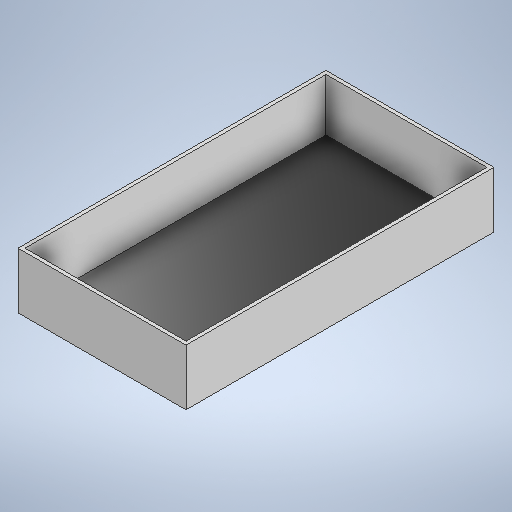
# Autodesk Inventor part: Blackout Box
Saved by Autodesk Inventor 2025 (Build 290162000, 162)
## iProperties
Created: 2024-06-19
Part Number: Blackout Box
Material: Generic
Document SubType Name: Modeling
Designer: User
Density: 1 g/cm^3
Appearance: Default
Author: User
Autodesk Inventor part; units mm, degrees
ref_plane "YZ Plane" through (0, 0, 0) normal (1, 0, 0) x (0, 1, 0)
ref_plane "XZ Plane" through (0, 0, 0) normal (0, 1, 0) x (-1, 0, 0)
ref_plane "XY Plane" through (0, 0, 0) normal (0, 0, 1) x (1, 0, 0)
sketch "Sketch1" plane through (0, 0, 0) normal (0, 1, 0) x (-1, 0, 0)
  line L0 (-152.4, 279.4) -> (152.4, 279.4)
  line L1 (152.4, 279.4) -> (152.4, -279.4)
  line L2 (152.4, -279.4) -> (-152.4, -279.4)
  line L3 (-152.4, -279.4) -> (-152.4, 279.4)
  line L4 (-152.4, 279.4) -> (152.4, -279.4) construction
  line L5 (152.4, 279.4) -> (-152.4, -279.4) construction
  line L6 (-146.05, 273.05) -> (146.05, 273.05)
  line L7 (146.05, 273.05) -> (146.05, -273.05)
  line L8 (146.05, -273.05) -> (-146.05, -273.05)
  line L9 (-146.05, -273.05) -> (-146.05, 273.05)
  line L10 (-146.05, 273.05) -> (146.05, -273.05) construction
  line L11 (146.05, 273.05) -> (-146.05, -273.05) construction
  point P0 (0, 0)
  dimension "d0" = 558.8
  dimension "d1" = 304.8
  dimension "d2" = 546.1
  dimension "d3" = 292.1
  constraints: 24 end point, 4 midpoint, 4 parallel, 2 horizontal, 2 perpendicular
  measures "d0" distance of L0.end L1.end
  measures "d1" distance of L1.end L2.end
  measures "d2" distance of L6.end L7.end
  measures "d3" distance of L7.end L8.end
extrude "Extrusion1" add sketch "Sketch1" along normal blind 6.35 contours L6 L7 L8 L9
extrude "Extrusion2" add sketch "Sketch1" along normal blind 101.6
sketch "Sketch2" plane through (0, 0, 0) normal (0, -1, 0) x (1, 0, 0)
  line L0 (-10, 50) -> (10, 50)
  line L1 (10, 50) -> (10, -50)
  line L2 (10, -50) -> (-10, -50)
  line L3 (-10, -50) -> (-10, 50)
  line L4 (-10, 50) -> (10, -50) construction
  line L5 (10, 50) -> (-10, -50) construction
  point P0 (0, 0)
  dimension "d8" = 100
  dimension "d9" = 20
  constraints: 12 end point, 2 midpoint, 2 parallel, 1 horizontal, 1 perpendicular
  measures "d8" distance of L0.end L1.end
  measures "d9" distance of L1.end L2.end
extrude "Extrusion3" add sketch "Sketch2" along normal blind 50
sketch "Sketch3" plane through (-10, 0, -50) normal (-1, 0, 0) x (0, 0, 1)
  line L0 (100, 0) -> (0, 0) projected
  line L1 (90, 0) -> (90, -40)
  line L2 (90, -40) -> (10, -40)
  line L3 (10, -40) -> (10, 0)
  line L4 (100, -50) -> (0, -50) projected
  line L5 (0, 0) -> (0, -50) projected
  line L6 (100, 0) -> (100, -50) projected
  point P0 (50, 0)
  dimension "d12" = 10
  dimension "d13" = 10
  dimension "d14" = 10
  constraints: 6 end point, 2 perpendicular, 2 point on line, 1 vertical
  measures "d12" distance between parallel lines of L4 L2
  measures "d13" distance between parallel lines of L5 L3
  measures "d14" distance between parallel lines of L6 L1
extrude "Extrusion4" cut sketch "Sketch3" against normal blind 50 contours L1 L2 L3 L0
body "Solid1"
